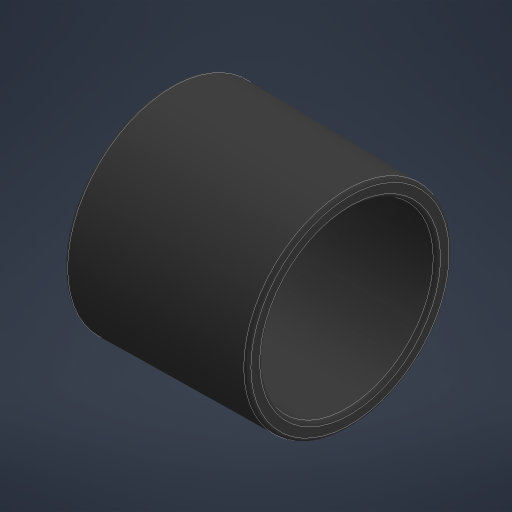
# Autodesk Inventor part: 12mm_Endcap
Saved by Autodesk Inventor 2024.1 (Build 281209000, 209)
## iProperties
Created: 2023-12-05
Part Number: 12mm_Endcap
Material: Rubber
Document SubType Name: Modeling
Designer: dzw04
Density: 0.93 g/cm^3
Appearance: Rubber - Black
Author: dzw04
Autodesk Inventor part; units mm, degrees
ref_plane "YZ Plane" through (0, 0, 0) normal (1, 0, 0) x (0, 1, 0)
ref_plane "XZ Plane" through (0, 0, 0) normal (0, 1, 0) x (-1, 0, 0)
ref_plane "XY Plane" through (0, 0, 0) normal (0, 0, 1) x (1, 0, 0)
sketch "Sketch1" plane through (0, 0, 0) normal (0, 1, 0) x (-1, 0, 0)
  line L0 (0, 0) -> (13, 0) construction
  line L1 (0.25, 6) -> (11, 6)
  line L2 (11, 6) -> (11, 0)
  line L3 (0, 6.25) -> (0, 6.8529)
  line L4 (13, 0) -> (13, 7.25) construction
  line L5 (12.2775, 7.2417) -> (0.2471, 7.1029)
  arc A0 (13, 0) -> (12.5284, 7.023) centre (-46.9979, -0.5017) ccw
  arc A1 (0.2471, 7.1029) -> (0, 6.8529) centre (0.25, 6.8529) ccw
  arc A2 (0, 6.25) -> (0.25, 6) centre (0.25, 6.25) ccw
  arc A3 (12.5284, 7.023) -> (12.2775, 7.2417) centre (12.2804, 6.9917) ccw
  line L6 (13, 0) -> (11, 0)
  point P0 (0, 6)
  point P1 (0, 7.1)
  point P2 (12.5, 7.2442)
  dimension "d0" = 13
  dimension "d1" = 11
  dimension "d2" = 6
  dimension "d3" = 1.1
  dimension "d5" = 2
  dimension "d6" = 7.25
  dimension "d7" = 60
  dimension "d8" = 0.5
  dimension "d9" = 0.25
  constraints: 14 end point, 9 point on circle, 7 point on line, 6 tangent, 4 centre point, 2 equal radius, 2 horizontal, 2 vertical, 1 collinear, 1 perpendicular
  measures "d0" distance of L0.end L0.start
  measures "d1" distance of point (0, 6) L1.end
  measures "d2" distance of L1.end L2.end
  measures "d3" distance of point (0, 6) point (0, 7.1)
  measures "d5" distance of L0.end L2.end
  measures "d6" distance of L0.end L4.end
  measures "d7" radius of A0
  measures "d8" horizontal distance of point (12.5, 7.244) L4.end
  measures "d9" radius of A1
revolve "Revolution1" add sketch "Sketch1" angle 360 about axis through (0, 0, 0) along (-1, 0, 0)
body "Solid1"
